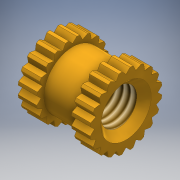
# Autodesk Inventor part: M3 Threaded Insert
Saved by Autodesk Inventor 2016 (Build 200138000, 138)
## iProperties
Created: 2017-02-03
Part Number: M3 Threaded Insert
Material: Brass, Soft Yellow, Welded
Document SubType Name: Modeling
Designer: Scott
Density: 8.5 g/cm^3
Appearance: Weld - Brass
Author: Scott
Autodesk Inventor part; units mm, degrees
ref_plane "YZ Plane" through (0, 0, 0) normal (1, 0, 0) x (0, 1, 0)
ref_plane "XZ Plane" through (0, 0, 0) normal (0, 1, 0) x (-1, 0, 0)
ref_plane "XY Plane" through (0, 0, 0) normal (0, 0, 1) x (1, 0, 0)
sketch "Sketch1" plane through (0, 0, 0) normal (0, 0, 1) x (1, 0, 0)
  line L0 (0, 0) -> (5.7743, 0) construction
  line L1 (0, 1.25) -> (5, 1.25)
  line L2 (5, 1.25) -> (5, 2.5)
  line L3 (5, 2.5) -> (3.7, 2.5)
  line L4 (3.7, 2.5) -> (3.7, 2)
  line L5 (3.7, 2) -> (1.3, 2)
  line L6 (1.3, 2) -> (1.3, 2.5)
  line L7 (1.3, 2.5) -> (0, 2.5)
  line L8 (0, 2.5) -> (0, 1.25)
  dimension "d0" = 1.25
  dimension "d1" = 1.3
  dimension "d2" = 1.3
  dimension "d3" = 5
  dimension "d4" = 2.5
  dimension "d5" = 2
  dimension "d6" = 5
  dimension "d7" = 0.7743
  constraints: 18 end point, 6 perpendicular, 2 horizontal, 2 point on line
  measures "d0" distance between parallel lines of L0 L1
  measures "d1" distance of L6.end L7.end
  measures "d2" distance of L2.end L3.end
  measures "d3" distance of L1.start L1.end
  measures "d4" distance between parallel lines of L0 L3
  measures "d5" distance between parallel lines of L0 L5
  measures "d6" distance from line of L0.start L2
  measures "d7" distance from line of L0.end L2
revolve "Revolution1" add sketch "Sketch1" angle 360 about axis through (0, 0, 0) along (1, 0, 0)
sketch "Sketch2" plane through (5, 0, 0) normal (1, 0, 0) x (0, 0, -1)
  line L0 (0, 0) -> (0, 3.0981) construction
  line L1 (0, 2.2) -> (0.5, 2.7)
  line L2 (0.5, 2.7) -> (-0.5, 2.7)
  line L3 (-0.5, 2.7) -> (0, 2.2)
  dimension "d9" = 2.2
  dimension "d10" = 45
  dimension "d11" = 45
  dimension "d12" = 0.5
  constraints: 8 end point, 1 perpendicular, 1 point on line, 1 vertical
  measures "d9" distance of L0.start L1.start
  measures "d10" angle of L0 L1
  measures "d11" angle of L0 L3
  measures "d12" distance from line of L1.start L2
extrude "Extrusion1" cut sketch "Sketch2" against normal through all
pattern_circular "Circular Pattern1" count 20 over 360 about axis through (2.5, 0, 0) along (1, 0, 0) of "Extrusion1"
chamfer "Chamfer1" distance 0.5 angle 45 2 edges at (5, -1.25, 0) (0, -1.25, 0)
thread "Thread1" size "M3x0.5" class "6H" standard "ANSI Metric M Profile" full length
body "Solid1"
